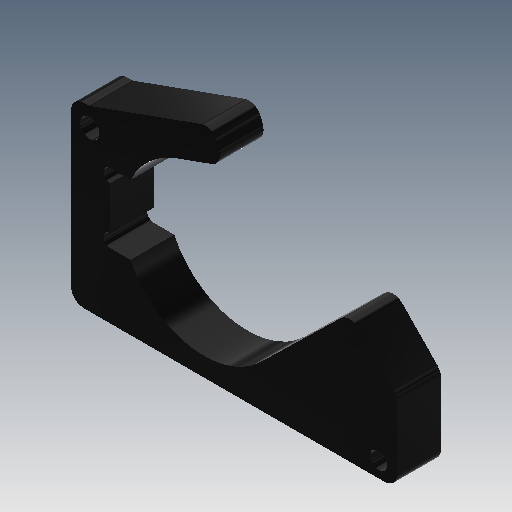
# Autodesk Inventor part: ジグ_1_2
Saved by Autodesk Inventor 2017.3 (Build 213256000, 256)
## iProperties
Created: 2016-05-31
Part Number: ジグ_1_2
Material: アセタール樹脂、黒
Document SubType Name: Modeling
Designer: hiroaki
Density: 1.425 g/cm^3
Appearance: 滑らか - 黒
Mass: 7.23258 g
Surface Area: 30.569 cm^2
Volume: 5.07549 cm^3
Author: hiroaki
Autodesk Inventor part; units mm, degrees
ref_plane "YZ Plane" through (0, 0, 0) normal (1, 0, 0) x (0, 1, 0)
ref_plane "XZ Plane" through (0, 0, 0) normal (0, 1, 0) x (-1, 0, 0)
ref_plane "XY Plane" through (0, 0, 0) normal (0, 0, 1) x (1, 0, 0)
derived "足首_独立ピッチ_1_1.ipt"
sketch "スケッチ1" plane through (0, 0, 0) normal (0, 0, 1) x (1, 0, 0)
  circle A0 centre (0, 0) radius 10.5 construction
  line L0 (0, 0) -> (-12, 0) construction
  arc A1 (0, 16) -> (-12, 10.583) centre (0, 0) ccw construction
  arc A2 (-12, -10.583) -> (0, -16) centre (0, 0) ccw construction
  line L1 (0, 16) -> (39.5, 16) construction
  line L2 (39.5, 16) -> (39.5, -16) construction
  line L3 (39.5, -16) -> (0, -16) construction
  circle A3 centre (-8.5, 0) radius 1.35
  circle A4 centre (0, 0) radius 8.5 construction
  line L4 (35.05, 121.7609) -> (35.05, 118.2391) construction
  line L5 (35.05, 118.2391) -> (32, 116.4782) construction
  line L6 (32, 116.4782) -> (28.95, 118.2391) construction
  line L7 (28.95, 118.2391) -> (28.95, 121.7609) construction
  line L8 (28.95, 121.7609) -> (32, 123.5218) construction
  line L9 (32, 123.5218) -> (35.05, 121.7609) construction
  line L10 (-12, -89.417) -> (-12, -110.583) construction
  line L11 (0, -84) -> (39.5, -84) construction
  line L12 (39.5, -84) -> (39.5, -116) construction
  line L13 (39.5, -116) -> (0, -116) construction
  arc A5 (0, -84) -> (-12, -89.417) centre (0, -100) ccw construction
  arc A6 (-12, -110.583) -> (0, -116) centre (0, -100) ccw construction
  line L14 (39.5, -89.5) -> (83, -89.5) construction
  line L15 (83, -89.5) -> (83, -110.5) construction
  line L16 (83, -110.5) -> (39.5, -110.5) construction
  line L17 (39.5, -110.5) -> (39.5, -89.5) construction
  line L18 (1, -86.5) -> (28, -86.5) construction
  line L19 (28, -86.5) -> (28, -113.5) construction
  line L20 (28, -113.5) -> (1, -113.5) construction
  line L21 (1, -113.5) -> (1, -86.5) construction
  circle A7 centre (1, -86.5) radius 1.35 construction
  circle A8 centre (1, -113.5) radius 1.35 construction
  circle A9 centre (28, -113.5) radius 1.35
  circle A10 centre (28, -86.5) radius 1.35 construction
  circle A11 centre (32, 20) radius 4.05
  circle A12 centre (32, 20) radius 4.05
  line L22 (10.583, 152) -> (-10.583, 152) construction
  line L23 (16, 140) -> (16, 100.5) construction
  line L24 (16, 100.5) -> (-16, 100.5) construction
  line L25 (-16, 100.5) -> (-16, 140) construction
  arc A13 (16, 140) -> (10.583, 152) centre (0, 140) ccw construction
  arc A14 (-10.583, 152) -> (-16, 140) centre (0, 140) ccw construction
  circle A15 centre (0, -100) radius 4.05 construction
  circle A16 centre (32, -80) radius 4.05 construction
  circle A17 centre (0, -100) radius 10.5 construction
  line L26 (32, -80) -> (0, -100) construction
  line L27 (45, -60.5) -> (77.5, -60.5) construction
  line L28 (77.5, -60.5) -> (77.5, -112) construction
  line L29 (77.5, -112) -> (45, -112) construction
  line L30 (45, -112) -> (45, -60.5) construction
  line L31 (45, -100) -> (77.5, -100) construction
  circle A18 centre (0, 140) radius 10.5 construction
  line L32 (-13.5, 139) -> (13.5, 139) construction
  line L33 (13.5, 139) -> (13.5, 112) construction
  line L34 (13.5, 112) -> (-13.5, 112) construction
  line L35 (-13.5, 112) -> (-13.5, 139) construction
  circle A19 centre (-13.5, 139) radius 1.35
  circle A20 centre (13.5, 139) radius 1.35
  circle A21 centre (-13.5, 112) radius 1.35
  circle A22 centre (13.5, 112) radius 1.35
  line L36 (-12, 10.583) -> (-12, -10.583) construction
  circle A23 centre (32, 20) radius 6.5 construction
  line L37 (32, 23.5218) -> (35.05, 21.7609) construction
  line L38 (35.05, 21.7609) -> (35.05, 18.2391) construction
  line L39 (35.05, 18.2391) -> (32, 16.4782) construction
  line L40 (32, 16.4782) -> (28.95, 18.2391) construction
  line L41 (28.95, 18.2391) -> (28.95, 21.7609) construction
  line L42 (28.95, 21.7609) -> (32, 23.5218) construction
  line L43 (21.5, 152) -> (61, 152) construction
  line L44 (61, 152) -> (61, 100.5) construction
  line L45 (61, 100.5) -> (21.5, 100.5) construction
  line L46 (21.5, 100.5) -> (21.5, 152) construction
  line L47 (21.5, 140) -> (61, 140) construction
  line L48 (16, 150.5) -> (66.5, 150.5) construction
  line L49 (66.5, 150.5) -> (66.5, 129.5) construction
  line L50 (66.5, 129.5) -> (16, 129.5) construction
  line L51 (16, 129.5) -> (16, 150.5) construction
  circle A24 centre (1, 13.5) radius 1.35
  circle A25 centre (1, -13.5) radius 1.35
  circle A26 centre (28, 13.5) radius 1.35
  circle A27 centre (28, -13.5) radius 1.35
  line L52 (1, 13.5) -> (1, -13.5) construction
  line L53 (1, -13.5) -> (28, -13.5) construction
  line L54 (1, 13.5) -> (28, 13.5) construction
  line L55 (28, 13.5) -> (28, -13.5) construction
  line L56 (0, 0) -> (1, 0) construction
  line L57 (32, 120) -> (32, 20) construction
  line L58 (0, 0) -> (0, 0) construction
  circle A28 centre (32, 120) radius 4.05
  line L59 (0, 140) -> (0, 40) construction
  circle A29 centre (0, 40) radius 4.05
  line L60 (0, 0) -> (0, -100) construction
  line L61 (32, 20) -> (32, -80) construction
  line L62 (0, 0) -> (0, 40) construction
  circle A30 centre (32, -80) radius 1.2 construction
  circle A31 centre (32, -80) radius 5 construction
  circle A32 centre (0, -100) radius 5.05 construction
  circle A33 centre (-8.5, -100) radius 1.35 construction
  circle A34 centre (0, -108.5) radius 1.35 construction
  circle A35 centre (8.5, -100) radius 1.35 construction
  circle A36 centre (0, -91.5) radius 1.35 construction
  line L63 (9.0705, -109.3127) -> (35.4886, -83.5818) construction
  arc A37 (-4.3963, -87.7659) -> (9.0705, -109.3127) centre (0, -100) ccw construction
  line L64 (0, 140) -> (0, 139) construction
  line L65 (0, 152) -> (0, 140) construction
  line L66 (-4.3963, -87.7659) -> (30.3091, -75.2946) construction
  arc A38 (35.4886, -83.5818) -> (30.3091, -75.2946) centre (32, -80) ccw construction
  circle A39 centre (-8.5, -100) radius 2.5 construction
  circle A40 centre (0, -100) radius 11 construction
  circle A41 centre (0, -100) radius 12 construction
  line L67 (-15, -94.5) -> (-12, -94.5) construction
  line L68 (-12, -94.5) -> (-12, -105.5) construction
  line L69 (-12, -105.5) -> (-15, -105.5) construction
  line L70 (-15, -105.5) -> (-15, -94.5) construction
  line L71 (-11.95, -94.45) -> (-15.05, -94.45)
  line L72 (-15.05, -94.45) -> (-15.05, -105.55)
  line L73 (-15.05, -105.55) -> (-11.95, -105.55)
  line L74 (-11.95, -105.55) -> (-11.95, -94.45)
  circle A42 centre (-15.05, -95.5) radius 1.05
  circle A43 centre (-11.95, -95.5) radius 1.05
  circle A44 centre (-15.05, -104.5) radius 1.05
  circle A45 centre (-11.95, -104.5) radius 1.05
  circle A46 centre (-18.3, -90.5) radius 1.55
  line L75 (-21.3, -87.5) -> (-21.3, -116)
  line L76 (-21.3, -116) -> (31, -116)
  line L77 (-21.3, -87.5) -> (-18.4414, -87.5)
  line L78 (-18.4414, -87.5) -> (1.4415, -80.3551)
  line L79 (1.4415, -80.3551) -> (3.1324, -85.0605)
  line L80 (3.1324, -85.0605) -> (-4.3963, -87.7659)
  line L81 (-4.3963, -87.7659) -> (-4.3963, -112.2341)
  arc A47 (-4.3963, -112.2341) -> (9.0705, -109.3127) centre (0, -100) ccw
  line L82 (9.0705, -109.3127) -> (23.3977, -95.3582)
  line L83 (23.3977, -95.3582) -> (31, -103.1635)
  circle A48 centre (0, -100) radius 16 construction
  line L84 (31, -103.1635) -> (31, -116)
  point P0 (-12, -100)
  point P1 (39.5, -100)
  point P2 (83, -100)
  point P3 (1, -100)
  point P4 (39.5, 0)
  point P5 (66.5, 140)
  point P6 (-15, -100)
  dimension "d5" = 2.1
  dimension "d1" = 12
  dimension "d2" = 11
  dimension "d3" = 3
  dimension "d4" = 0.05
  dimension "d6" = 3.1
  dimension "d7" = 3.3
  dimension "d8" = 4
  dimension "d11" = 3
  dimension "d12" = 5
  dimension "d13" = 8
  dimension "d14" = 20
  dimension "d15" = 3
  dimension "d16" = 3
  dimension "d22" = 3
  measures "d1" distance from line of A40.centre L68
  measures "d2" distance of L69.end L67.start
  measures "d3" distance of L67.start L67.end
  measures "d4" distance between parallel lines of L71 L67
  measures "d6" diameter of A46
  measures "d7" distance from line of L70 A46.centre
  measures "d8" distance from line of L67 A46.centre
  measures "d11" distance from line of A46.centre L75
  measures "d12" distance of L78.end L79.end
  measures "d13" distance from line of A40.centre L79
  measures "d14" distance from line of A40.centre L83
  measures "d15" distance from line of A46.centre L77
  measures "d16" radial gap between concentric circles of A48 A37
  measures "d22" distance between parallel lines of L84 L19
extrude "押し出し1" add sketch "スケッチ1" along normal blind 7 contours L77 L78 L79 L80 L81 A47 L82 L83 L84 L76 L75
sketch "スケッチ3" plane through (-21.3, -116, 7) normal (0, 0, 1) x (1, 0, 0)
  arc A0 (16.9037, 3.7659) -> (30.3705, 6.6873) centre (21.3, 16) ccw projected
  circle A1 centre (21.3, 16) radius 13
  point P0 (21.3, 116)
  constraints: 1 centre point, 1 coincident, 1 concentric
extrude "押し出し2" cut sketch "スケッチ3" against normal blind 10
fillet "フィレット1" radius 2 8 edges at (1.4415, -80.3551, 3.5) (3.1324, -85.0605, 3.5) (23.3977, -95.3582, 3.5) (31, -103.1635, 3.5) (31, -116, 3.5) (-21.3, -116, 3.5) (-21.3, -87.5, 3.5) (-18.4414, -87.5, 3.5)
equation "\"d11\" = d9"
equation "\"d9\" = 3"
